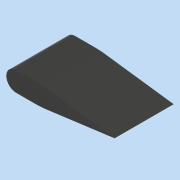
# Autodesk Inventor part: foreDivePlanes
Saved by Autodesk Inventor 2017 (Build 210142000, 142)
## iProperties
Created: 2016-12-09
Part Number: foreDivePlanes
Material: ABS Plastic
Document SubType Name: Modeling
Designer: techn
Density: 1.06 g/cm^3
Appearance: Smooth - Black
Author: techn
Autodesk Inventor part; units mm, degrees
ref_plane "YZ Plane" through (0, 0, 0) normal (1, 0, 0) x (0, 1, 0)
ref_plane "XZ Plane" through (0, 0, 0) normal (0, 1, 0) x (-1, 0, 0)
ref_plane "XY Plane" through (0, 0, 0) normal (0, 0, 1) x (1, 0, 0)
sketch "Sketch5" plane through (0, 0, 0) normal (0, 0, 1) x (1, 0, 0)
  circle A0 centre (0, 0) radius 3.175
  line L0 (0, 3.175) -> (7.9375, 3.175)
  line L1 (0, -3.175) -> (7.9375, -3.175)
  line L2 (7.9375, 3.175) -> (31.75, 0)
  line L3 (31.75, 0) -> (7.9375, -3.175)
  dimension "d16" = 6.35
  dimension "d17" = 7.9375
  dimension "d18" = 7.9375
  dimension "d19" = 31.75
  constraints: 8 end point, 2 horizontal, 2 point on circle, 2 tangent, 1 centre point, 1 coincident
  measures "d16" diameter of A0
  measures "d17" distance of L0.start L0.end
  measures "d18" distance of L1.start L1.end
  measures "d19" distance of L2.end point (0, 0)
extrude "Extrusion2" add sketch "Sketch5" along normal blind 19.05
sketch "Sketch6" plane through (0, 0, 0) normal (0, 0, -1) x (-1, 0, 0)
  circle A0 centre (0, 0) radius 1.5875
  dimension "d22" = 3.175
  constraints: 1 centre point, 1 coincident
  measures "d22" diameter of A0
sketch "Sketch7" plane through (0, 0, 0) normal (0, 1, 0) x (-1, 0, 0)
  line L0 (0, 0) -> (0, 3.175)
  line L1 (-7.9375, 11.1125) -> (-8.763, 11.1125)
  arc A0 (0, 3.175) -> (-7.9375, 11.1125) centre (-7.9375, 3.175) ccw
  dimension "d23" = 3.175
  dimension "d26" = 0.8255
  dimension "d27" = 7.9375
  dimension "d28" = 7.9375
  constraints: 4 end point, 2 point on circle, 1 centre point, 1 tangent, 1 vertical
  measures "d23" distance of L0.start L0.end
  measures "d26" distance of L1.start L1.end
  measures "d27" horizontal distance of L1.start L0.end
  measures "d28" horizontal distance of L1.start L0.end
sweep "Sweep2" cut profiles "Sketch6" path "Sketch7" path curves L0 A0 L1
fillet "Fillet1" radius 25.4 2 edges at (7.9375, 3.175, 9.525) (7.9375, -3.175, 9.525)
body "Solid2"
